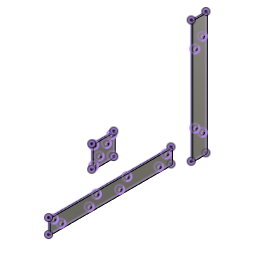
Chassis frame v2 (Autodesk Fusion 360 design; units mm, degrees)
Autodesk Fusion 360 part; units mm, degrees
sketch "Design sketch" plane through (0, 0, 0) normal (1, 0, 0) x (0, 1, 0)
  line L0 (125, 15) -> (-125, 15)
  line L1 (-125, 15) -> (-125, -15)
  line L2 (-125, -15) -> (125, -15)
  line L3 (125, -15) -> (125, 15)
  circle A0 centre (-100, -7.5) radius 1.75
  line L4 (196.3649, 218.9658) -> (166.3649, 218.9658)
  line L5 (166.3649, 218.9658) -> (166.3649, -31.0342)
  line L6 (196.3649, -31.0342) -> (196.3649, 218.9658)
  circle A1 centre (-115, 7.5) radius 1.75
  line L7 (166.3649, -31.0342) -> (196.3649, -31.0342)
  circle A2 centre (100, -7.5) radius 1.75
  circle A3 centre (115, 7.5) radius 1.75
  circle A4 centre (173.8649, 23.9658) radius 1.75
  circle A5 centre (188.8649, 8.9658) radius 1.75
  circle A6 centre (173.8649, 163.9658) radius 1.75
  circle A7 centre (188.8649, 178.9658) radius 1.75
  line L8 (-36.8557, 56.4397) -> (8.1443, 56.4397)
  line L9 (8.1443, 56.4397) -> (8.1443, 101.4397)
  line L10 (8.1443, 101.4397) -> (-36.8557, 101.4397)
  line L11 (-36.8557, 101.4397) -> (-36.8557, 56.4397)
  circle A8 centre (-32.8557, 60.4397) radius 1.75
  circle A9 centre (-32.8557, 97.4397) radius 1.75
  circle A10 centre (4.1443, 60.4397) radius 1.75
  circle A11 centre (4.1443, 97.4397) radius 1.75
  circle A12 centre (35, 7.5) radius 1.75
  circle A13 centre (20, -7.5) radius 1.75
  circle A14 centre (-42.3535, -7.313) radius 1.75
  circle A15 centre (-27.3535, 7.687) radius 1.75
  circle A16 centre (-21.8921, 72.2799) radius 1.75
  circle A17 centre (-6.8921, 87.2799) radius 1.75
  point P0 (20, -7.5)
  dimension "d1" = 250
  dimension "d2" = 30
  dimension "d8" = 3.5
  dimension "d30" = 3.5
  dimension "d49" = 3.5
  dimension "d50" = 3.5
  dimension "d53" = 15
  dimension "d66" = 15
  dimension "d67" = 15
  dimension "d68" = 3.5
  dimension "d69" = 3.5
  dimension "d75" = 15
  dimension "d78" = 30
  dimension "d79" = 250
  dimension "d83" = 15
  dimension "d84" = 15
  dimension "d85" = 3.5
  dimension "d86" = 3.5
  dimension "d87" = 15
  dimension "d89" = 15
  dimension "d92" = 10
  dimension "d93" = 10
  dimension "d94" = 40
  dimension "d95" = 40
  dimension "d96" = 7.5
  dimension "d98" = 7.5
  dimension "d99" = 7.5
  dimension "d100" = 7.5
  dimension "d101" = 45
  dimension "d102" = 45
  dimension "d103" = 3.5
  dimension "d104" = 3.5
  dimension "d105" = 3.5
  dimension "d106" = 3.5
  dimension "d107" = 4
  dimension "d108" = 4
  dimension "d109" = 4
  dimension "d110" = 4
  dimension "d111" = 4
  dimension "d112" = 4
  dimension "d113" = 4
  dimension "d114" = 4
  dimension "d115" = 3.5
  dimension "d116" = 15
  dimension "d117" = 15
  dimension "d118" = 7.5
  dimension "d119" = 3.5
  dimension "d120" = 3.5
  dimension "d121" = 3.5
  dimension "d122" = 3.5
  dimension "d123" = 3.5
  constraint horizontal L0
  constraint perpendicular L0 L1
  constraint parallel L0 L2
  constraint parallel L1 L3
  constraint horizontal L4
  constraint perpendicular L4 L5
  constraint parallel L4 L7
  constraint parallel L5 L6
  constraint horizontal L8
  constraint vertical L9
  constraint horizontal L10
  constraint vertical L11
  constraint coincident P0 A13.centre
  measures "d1" distance of L1.end L2.end
  measures "d2" distance of L0.end L1.end
  measures "d8" diameter of A0
  measures "d30" diameter of A1
  measures "d49" diameter of A2
  measures "d50" diameter of A3
  measures "d53" horizontal distance of A2.centre A3.centre
  measures "d66" vertical distance of A0.centre A1.centre
  measures "d67" horizontal distance of A0.centre A1.centre
  measures "d68" diameter of A4
  measures "d69" diameter of A5
  measures "d75" vertical distance of A2.centre A3.centre
  measures "d78" distance of L5.end L6.start
  measures "d79" distance of L4.start L6.start
  measures "d83" horizontal distance of A4.centre A5.centre
  measures "d84" vertical distance of A4.centre A5.centre
  measures "d85" diameter of A6
  measures "d86" diameter of A7
  measures "d87" horizontal distance of A6.centre A7.centre
  measures "d89" vertical distance of A6.centre A7.centre
  measures "d92" distance of L3 A3.centre
  measures "d93" distance of L1 A1.centre
  measures "d94" distance of L7 A5.centre
  measures "d95" distance of L4 A7.centre
  measures "d96" distance of L2 A2.centre
  measures "d98" distance of L5 A4.centre
  measures "d99" distance of L2 A0.centre
  measures "d100" distance of L5 A6.centre
  measures "d101" distance of L8.start L8.end
  measures "d102" distance of L8.start L10.end
  measures "d103" diameter of A8
  measures "d104" diameter of A9
  measures "d105" diameter of A10
  measures "d106" diameter of A11
  measures "d107" distance of L9 A10.centre
  measures "d108" distance of L8 A10.centre
  measures "d109" distance of L8 A8.centre
  measures "d110" distance of L11 A8.centre
  measures "d111" distance of L10 A9.centre
  measures "d112" distance of L11 A9.centre
  measures "d113" distance of L10 A11.centre
  measures "d114" distance of L9 A11.centre
  measures "d115" diameter of A12
  measures "d116" horizontal distance of P0 A12.centre
  measures "d117" vertical distance of P0 A12.centre
  measures "d118" distance of L2 P0
  measures "d119" diameter of A13
  measures "d120" diameter of A15
  measures "d121" diameter of A14
  measures "d122" diameter of A17
  measures "d123" diameter of A16
extrude "Extrude5" add sketch "Design sketch" along normal blind 3 makes body 1 at (0, -61.951, 3.6963) makes body 2 at (0, 183.6225, 206.1631) makes body 3 at (0, -8.014, 73.1482)
sketch "Laser cut ready sketh" plane through (0, 0, 0) normal (1, 0, 0) x (0, 0, -1)
  circle A0 centre (7.313, -42.3535) radius 1.75
  circle A1 centre (-7.687, -27.3535) radius 1.75
  circle A2 centre (7.5, 20) radius 1.75
  circle A3 centre (-7.5, 115) radius 1.75
  circle A4 centre (7.5, 100) radius 1.75
  circle A5 centre (7.5, -100) radius 1.75
  circle A6 centre (-7.5, 35) radius 1.75
  circle A7 centre (-7.5, -115) radius 1.75
  line L0 (15, -125) -> (15, 125)
  line L1 (-15, -125) -> (15, -125)
  line L2 (-15, 125) -> (-15, -125)
  line L3 (15, 125) -> (-15, 125)
  circle A8 centre (-72.2799, -21.8921) radius 1.75
  circle A9 centre (-97.4397, 4.1443) radius 1.75
  circle A10 centre (-60.4397, 4.1443) radius 1.75
  circle A11 centre (-87.2799, -6.8921) radius 1.75
  circle A12 centre (-97.4397, -32.8557) radius 1.75
  circle A13 centre (-60.4397, -32.8557) radius 1.75
  line L4 (-101.4397, 8.1443) -> (-101.4397, -36.8557)
  line L5 (-56.4397, 8.1443) -> (-101.4397, 8.1443)
  line L6 (-56.4397, -36.8557) -> (-56.4397, 8.1443)
  line L7 (-101.4397, -36.8557) -> (-56.4397, -36.8557)
  circle A14 centre (-178.9658, 188.8649) radius 1.75
  circle A15 centre (-163.9658, 173.8649) radius 1.75
  circle A16 centre (-23.9658, 173.8649) radius 1.75
  circle A17 centre (-8.9658, 188.8649) radius 1.75
  line L8 (-218.9658, 166.3649) -> (31.0342, 166.3649)
  line L9 (-218.9658, 196.3649) -> (-218.9658, 166.3649)
  line L10 (31.0342, 196.3649) -> (-218.9658, 196.3649)
  line L11 (31.0342, 166.3649) -> (31.0342, 196.3649)
extrude "Extrude2" [suppressed]
equation "d1 = partLength"
equation "d2 = partWidth"
equation "partLength = 250 mm"
equation "partWidth = 30 mm"
equation "boltHole = 3.5 mm"
equation "d8 = boltHole"
equation "boltTriangleHeight = 7 mm"
equation "boltFromEdgesClose = 10 mm"
equation "boltGap = 15 mm"
equation "d30 = boltHole"
equation "boltFromEdgesFar = 40 mm"
equation "d49 = boltHole"
equation "d50 = boltHole"
equation "d53 = boltGap"
equation "d66 = boltGap"
equation "d67 = boltGap"
equation "d68 = boltHole"
equation "d69 = boltHole"
equation "d75 = boltGap"
equation "d78 = partWidth"
equation "d79 = partLength"
equation "d83 = boltGap"
equation "d84 = boltGap"
equation "d85 = boltHole"
equation "d86 = boltHole"
equation "d87 = boltGap"
equation "d89 = boltGap"
equation "d92 = boltFromEdgesClose"
equation "d93 = boltFromEdgesClose"
equation "d94 = boltFromEdgesFar"
equation "d95 = boltFromEdgesFar"
equation "d96 = ( partWidth - boltGap ) / 2"
equation "boltGapFromSide = ( partWidth - boltGap ) / 2"
equation "d98 = boltGapFromSide"
equation "d99 = boltGapFromSide"
equation "d100 = boltGapFromSide"
equation "d107 = ( ( 45 - 37 ) / 2 ) * 1 mm"
equation "d108 = ( ( 45 - 37 ) / 2 ) * 1 mm"
equation "d109 = ( ( 45 - 37 ) / 2 ) * 1 mm"
equation "d110 = ( ( 45 - 37 ) / 2 ) * 1 mm"
equation "d111 = ( ( 45 - 37 ) / 2 ) * 1 mm"
equation "d112 = ( ( 45 - 37 ) / 2 ) * 1 mm"
equation "d113 = ( ( 45 - 37 ) / 2 ) * 1 mm"
equation "d114 = ( ( 45 - 37 ) / 2 ) * 1 mm"
equation "d115 = boltHole"
equation "d116 = boltGap"
equation "d117 = boltGap"
equation "d118 = boltGapFromSide"
equation "d119 = boltHole"
equation "d120 = boltHole"
equation "d121 = boltHole"
equation "d122 = boltHole"
equation "d123 = boltHole"
